sensor_holder_thing (Autodesk Fusion 360 design; units mm, degrees)
Autodesk Fusion 360 part; units mm, degrees
sketch "Sketch1" plane through (0, 0, 0) normal (0, 0, 1) x (1, 0, 0)
  line L0 (0, 0) -> (-3.7585, 6.5099)
  line L1 (-3.7585, 6.5099) -> (0, 13.0198)
  line L2 (0, 13.0198) -> (7.517, 13.0198)
  line L3 (7.517, 13.0198) -> (11.2755, 6.5099)
  line L4 (11.2755, 6.5099) -> (7.517, 0)
  line L5 (7.517, 0) -> (0, 0)
  dimension "d1" = 120
  dimension "d2" = 120
  dimension "d3" = 7.517
  dimension "d4" = 7.517
  dimension "d5" = 7.517
  dimension "d6" = 7.517
  constraint coincident L0.start L5.end
  constraint horizontal L2
  constraint parallel L2 L5
  constraint parallel L1 L4
  constraint parallel L0 L3
  measures "d1" angle of L4 L5
  measures "d2" angle of L0 L5
  measures "d3" distance of L3.end L4.end
  measures "d4" distance of L4.end L0.start
  measures "d5" distance of L0.start L0.end
  measures "d6" distance of L2.end L3.end
extrude "Extrude1" add sketch "Sketch1" along normal blind 14 draft 1.1
sketch "Sketch2" plane through (0, 0, 14) normal (0, 0, 1) x (-1, 0, 0)
  line L0 (0.1552, 0.2688) -> (-7.6722, 0.2688)
  line L1 (-7.6722, 0.2688) -> (-11.5859, -6.5099)
  line L2 (-11.5859, -6.5099) -> (-7.6722, -13.2886)
  line L3 (-7.6722, -13.2886) -> (0.1552, -13.2886)
  line L4 (0.1552, -13.2886) -> (4.0689, -6.5099)
  line L5 (4.0689, -6.5099) -> (0.1552, 0.2688)
  line L6 (0.1552, -13.2886) -> (-7.6722, 0.2688)
  line L7 (4.0689, -6.5099) -> (-11.5859, -6.5099)
  line L8 (-7.6722, -13.2886) -> (0.1552, 0.2688)
  circle A0 centre (-3.7585, -6.5099) radius 19
  circle A1 centre (-3.7585, -6.5099) radius 21.3499
  line L9 (5.0153, -25.9737) -> (5.8455, -26.0477)
  line L10 (4.3962, -24.2552) -> (5.1351, -23.2999)
  line L11 (-3.7585, -6.5099) -> (-3.7585, -7)
  line L12 (-13.3271, -26.7079) -> (-13.2828, -26.7025)
  line L13 (-12.3737, -24.5944) -> (-12.4136, -24.5402)
  line L14 (-3.7585, -6.5099) -> (-25.1084, -6.5099)
  line L15 (-3.7585, -6.5099) -> (-14.4334, -24.9995)
  arc A2 (-13.2585, -22.9644) -> (-14.4334, -24.9995) centre (-13.846, -23.9819) ccw
  arc A3 (-25.1084, -6.5099) -> (-22.7585, -6.5099) centre (-23.9334, -6.5099) ccw
  line L16 (-11.5859, -6.5099) -> (-0.7542, 12.2511)
  line L17 (-7.6722, -13.2886) -> (13.9911, -13.2886)
  dimension "d9" = 38
  dimension "d10" = 2.3499
  constraint coincident L3.end L4.start
  constraint coincident L0.end L1.start
  constraint coincident L1.end L2.start
  constraint coincident L0.start L5.end
  constraint coincident L4.end L5.start
  constraint coincident L2.end L3.start
  constraint midpoint L8 A0.centre
  constraint coincident A1 L9.start
  constraint coincident A0 L10.end
  constraint coincident A0.centre A1.centre
  constraint vertical L11
  constraint coincident A1 L14.end
  constraint coincident A1 L15.end
  constraint coincident L15 A2.start
  constraint coincident A0 A2.start
  constraint coincident L14 A3.end
  constraint coincident A0 A3.end
  constraint coincident L14 A3.centre
  constraint coincident L15 A2.centre
  constraint collinear L8 L15
  constraint collinear L7 L14
  constraint coincident A0 L16.end
  constraint parallel L1 L16
  constraint coincident A0 L17.end
  constraint horizontal L17
  measures "d9" diameter of A0
extrude "Extrude2" add sketch "Sketch2" along normal blind 1.5 contours L0 L6 L8 | L0 L4 L5 A0 L16 L17 | L5 L7 L8 | L1 L6 L7 L14 L16 | L4 L6 L7 | L2 L7 L8 L14 L15 | L3 L6 L8 L15 L17 | A0 A1 L14 L15 | L14 A3 | L15 A2
extrude "Extrude3" add sketch "Sketch2" along normal blind 14.5 contours A0 A1 L14 L15 | L14 A3 | L15 A2
equation "d2 = d1"
equation "d4 = d3"
equation "d5 = d3"
equation "d6 = d3"
